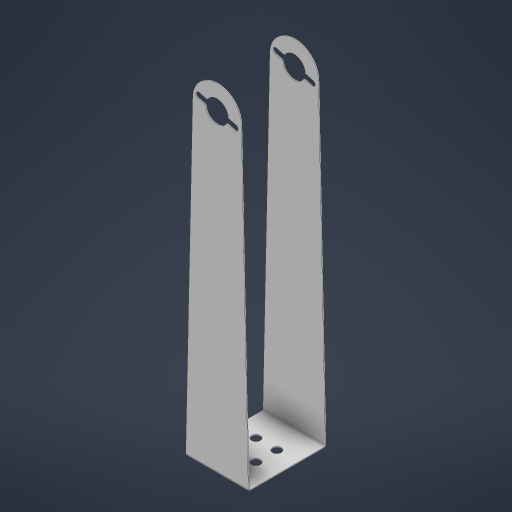
# Autodesk Inventor part: SoporteH
Saved by Autodesk Inventor 2024 (Build 280153000, 153)
## iProperties
Created: 2023-05-12
Part Number: SoporteH
Material: Genérico
Document SubType Name: Sheet Metal
Designer: javie
Density: 1 g/cm^3
Sheet Metal Rule: Por defecto_mm
Appearance: Valor por defecto
Author: javie
Autodesk Inventor part; units mm, degrees
ref_plane "YZ Plane" through (0, 0, 0) normal (1, 0, 0) x (0, 1, 0)
ref_plane "XZ Plane" through (0, 0, 0) normal (0, 1, 0) x (-1, 0, 0)
ref_plane "XY Plane" through (0, 0, 0) normal (0, 0, 1) x (1, 0, 0)
sketch "Boceto1" plane through (0, 0, 0) normal (0, 1, 0) x (-1, 0, 0)
  line L0 (18, 22) -> (-18, 22)
  line L1 (-18, 22) -> (-18, -22)
  line L2 (-18, -22) -> (18, -22)
  line L3 (18, -22) -> (18, 22)
  line L4 (18, -22) -> (-18, -22)
  arc A0 (-14, -202) -> (14, -202) centre (0, -202) ccw
  circle A1 centre (6, 6) radius 2.5
  circle A2 centre (-6, 6) radius 2.5
  circle A3 centre (-6, -6) radius 2.5
  circle A4 centre (6, -6) radius 2.5
  arc A5 (6.4147, -202.0624) -> (-5.5865, -198.8467) centre (0, -202) ccw
  arc A6 (10.1145, -206.3666) -> (10.9427, -203.2756) centre (10.5286, -204.8211) ccw
  arc A7 (10.1145, -206.3666) -> (10.9427, -203.2756) centre (10.5286, -204.8211) ccw
  arc A8 (-10.1145, -197.6334) -> (-10.9427, -200.7244) centre (-10.5286, -199.1789) ccw
  arc A9 (-10.1145, -197.6334) -> (-10.9427, -200.7244) centre (-10.5286, -199.1789) ccw
  line L5 (10.1145, -206.3666) -> (5.5865, -205.1533)
  line L6 (10.1145, -206.3666) -> (5.5865, -205.1533)
  line L7 (6.4147, -202.0624) -> (10.9427, -203.2756)
  line L8 (10.9427, -203.2756) -> (6.4147, -202.0624)
  line L9 (-6.4147, -201.9376) -> (-10.9427, -200.7244)
  line L10 (-10.9427, -200.7244) -> (-6.4147, -201.9376)
  line L11 (-10.1145, -197.6334) -> (-5.5865, -198.8467)
  line L12 (-5.5865, -198.8467) -> (-10.1145, -197.6334)
  arc A10 (6.4147, -202.0624) -> (-5.5865, -198.8467) centre (0, -202) ccw
  arc A11 (-6.4147, -201.9376) -> (5.5865, -205.1533) centre (0, -202) ccw
  line L13 (14, -202) -> (18, -22)
  line L14 (-14, -202) -> (-18, -22)
  line L15 (26.544, 0) -> (-28.5173, 0)
  arc A12 (14, 202) -> (-14, 202) centre (0, 202) ccw
  arc A13 (-5.5865, 198.8467) -> (6.4147, 202.0624) centre (0, 202) ccw
  arc A14 (10.9427, 203.2756) -> (10.1145, 206.3666) centre (10.5286, 204.8211) ccw
  arc A15 (10.9427, 203.2756) -> (10.1145, 206.3666) centre (10.5286, 204.8211) ccw
  arc A16 (-10.9427, 200.7244) -> (-10.1145, 197.6334) centre (-10.5286, 199.1789) ccw
  arc A17 (-10.9427, 200.7244) -> (-10.1145, 197.6334) centre (-10.5286, 199.1789) ccw
  line L16 (10.1145, 206.3666) -> (5.5865, 205.1533)
  line L17 (10.1145, 206.3666) -> (5.5865, 205.1533)
  line L18 (6.4147, 202.0624) -> (10.9427, 203.2756)
  line L19 (10.9427, 203.2756) -> (6.4147, 202.0624)
  line L20 (-6.4147, 201.9376) -> (-10.9427, 200.7244)
  line L21 (-10.9427, 200.7244) -> (-6.4147, 201.9376)
  line L22 (-10.1145, 197.6334) -> (-5.5865, 198.8467)
  line L23 (-5.5865, 198.8467) -> (-10.1145, 197.6334)
  arc A18 (-5.5865, 198.8467) -> (6.4147, 202.0624) centre (0, 202) ccw
  arc A19 (5.5865, 205.1533) -> (-6.4147, 201.9376) centre (0, 202) ccw
  line L24 (14, 202) -> (18, 22)
  line L25 (-14, 202) -> (-18, 22)
  point P0 (0, 0)
  dimension "d3" = 18
  dimension "d7" = 5
  dimension "d8" = 6
  dimension "d9" = 6
  dimension "d12" = 360
  dimension "d14" = 14
  dimension "d15" = 180
  constraints: 52 end point, 32 point on circle, 20 centre point, 19 symmetric about line, 6 coincident, 5 equal length, 4 tangent, 3 horizontal, 1 perpendicular, 17 other
  measures "d3" distance from line of point (0, 0) L3
  measures "d7" diameter of A1
  measures "d8" horizontal distance of point (0, 0) A1.centre
  measures "d9" horizontal distance of A1.centre point (0, 0)
  measures "d14" radius of A0
  measures "d15" distance from line of L2 A0.centre
extrude "Placa1" add sketch "Boceto1" along normal blind 0.5
fold "Pliegue1" angle 90 bend radius 0.5 thickness 0.5 k factor 0.44 line from (18, 0, -22) to (-18, 0, -22) line at bend centre moving side (0, 0, -1) folds toward (0, 1, 0)
fold "Pliegue2" angle 90 bend radius 0.5 thickness 0.5 k factor 0.44 line from (-18, 0, 22) to (18, 0, 22) line at bend centre moving side (0, 0, 1) folds toward (0, 1, 0)
equation "\"d16\" = Grosor"
equation "\"d17\" = Anchura_desahogo_plegado"
equation "\"d18\" = Profundidad_desahogo_plegado"
equation "\"d19\" = Remanente_mínimo"
equation "\"d20\" = Radiodetransición"
equation "\"d22\" = Radio_pliegue"
equation "\"d23\" = Anchura_desahogo_plegado"
equation "\"d24\" = Profundidad_desahogo_plegado"
equation "\"d25\" = Remanente_mínimo"
equation "\"d26\" = Radiodetransición"
equation "\"d28\" = Radio_pliegue"
equation "\"Radio_pliegue\" = Grosor"
equation "\"Anchura_desahogo_plegado\" = Grosor"
equation "\"Profundidad_desahogo_plegado\" = 0.5 * Grosor"
equation "\"Tamaño_destalonado\" = 4 * Grosor"
equation "\"Remanente_mínimo\" = 2 * Grosor"
equation "\"Radiodetransición\" = Radio_pliegue"
equation "\"Tamaño_de_radio_de_Jacobi\" = Radio_pliegue"
equation "\"TamañoSeparación\" = Grosor"
equation "\"Grosor\" = 0.5"
